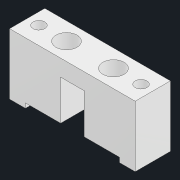
# Autodesk Inventor part: scara-base7
Saved by Autodesk Inventor 2022 (Build 260153000, 153)
## iProperties
Created: 2021-10-21
Part Number: scara-base7
Material: ABS プラスチック
Document SubType Name: Modeling
Designer: Yuta Kage
Density: 1.06 g/cm^3
Appearance: 滑らか - 白
Author: Yuta Kage
Autodesk Inventor part; units mm, degrees
ref_plane "YZ Plane" through (0, 0, 0) normal (1, 0, 0) x (0, 1, 0)
ref_plane "XZ Plane" through (0, 0, 0) normal (0, 1, 0) x (-1, 0, 0)
ref_plane "XY Plane" through (0, 0, 0) normal (0, 0, 1) x (1, 0, 0)
sketch "スケッチ1" plane through (0, 0, 0) normal (0, 0, 1) x (1, 0, 0)
  line L0 (-26.75, 0) -> (26.75, 0)
  line L1 (26.75, 0) -> (26.75, -26)
  line L2 (5, -24) -> (5, -7)
  line L3 (5, -7) -> (-5, -7)
  line L4 (-5, -7) -> (-5, -24)
  line L5 (-26.75, -26) -> (-26.75, 0)
  line L6 (-26.75, -26) -> (-20, -26)
  line L7 (-20, -26) -> (-20, -24)
  line L8 (-20, -24) -> (-5, -24)
  line L9 (5, -24) -> (20, -24)
  line L10 (20, -24) -> (20, -26)
  line L11 (20, -26) -> (26.75, -26)
  point P0 (0, 0)
  dimension "d0" = 53.5
  dimension "d1" = 10
  dimension "d2" = 5
  dimension "d3" = 26.75
  dimension "d4" = 40
  dimension "d5" = 20
  dimension "d6" = 17
  dimension "d7" = 2
  dimension "d29" = 24
  constraints: 24 end point, 10 perpendicular, 2 horizontal, 2 horizontal alignment, 1 midpoint
  measures "d0" distance of L0.start L0.end
  measures "d1" distance of L2.end L3.end
  measures "d2" distance from line of point (0, 0) L4
  measures "d3" distance from line of point (0, 0) L5
  measures "d4" distance between parallel lines of L10 L7
  measures "d5" distance from line of point (0, 0) L7
  measures "d6" distance between parallel lines of L8 L3
  measures "d7" distance of L9.end L10.end
  measures "d29" distance between parallel lines of L0 L9
extrude "押し出し1" add sketch "スケッチ1" along normal mid plane 15
sketch "スケッチ2" plane through (-26.75, 0, 7.5) normal (0, 1, 0) x (1, 0, 0)
  point P0 (26.75, 7.5)
  point P1 (16.75, 7.5)
  point P2 (36.75, 7.5)
  dimension "d11" = 10
  dimension "d12" = 10
  constraints: 2 horizontal alignment
  measures "d11" distance of point (26.75, 7.5) point (36.75, 7.5)
  measures "d12" distance of point (16.75, 7.5) point (26.75, 7.5)
hole "穴1" at (-10, 0, 0) at (10, 0, 0) direction (0, -1, 0) diameter 5.5 end through all counterbore diameter 9 counterbore depth 8 clearance for "Socket Head Cap Screw" size "M5" standard "Ansi Metric M Profile"
sketch "スケッチ3" plane through (-26.75, 0, 7.5) normal (0, 1, 0) x (1, 0, 0)
  point P0 (26.75, 7.5)
  point P1 (5, 7.5)
  point P2 (48.5, 7.5)
  dimension "d20" = 21.75
  dimension "d21" = 21.75
  constraints: 2 horizontal alignment
  measures "d20" distance of point (26.75, 7.5) point (48.5, 7.5)
  measures "d21" distance of point (5, 7.5) point (26.75, 7.5)
hole "穴2" at (-21.75, 0, 0) at (21.75, 0, 0) direction (0, -1, 0) diameter 5 depth 6 tip angle 118
equation "\"d2\" = 0.5 * d1"
equation "\"d3\" = 0.5 * d0"
equation "\"d5\" = 0.5 * d4"
equation "\"d12\" = d11"
equation "\"d21\" = d20"
